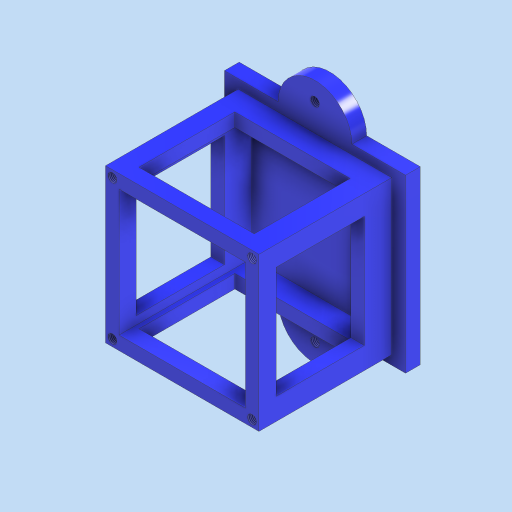
# Autodesk Inventor part: Base para Driver Corregida
Saved by Autodesk Inventor 2024 (Build 280153000, 153)
## iProperties
Created: 2023-12-03
Part Number: Base para Driver Corregida
Material: Genérico
Document SubType Name: Modeling
Designer: R3PT1L
Density: 1 g/cm^3
Appearance: Valor por defecto
Author: R3PT1L
Autodesk Inventor part; units mm, degrees
ref_plane "YZ Plane" through (0, 0, 0) normal (1, 0, 0) x (0, 1, 0)
ref_plane "XZ Plane" through (0, 0, 0) normal (0, 1, 0) x (-1, 0, 0)
ref_plane "XY Plane" through (0, 0, 0) normal (0, 0, 1) x (1, 0, 0)
sketch "Boceto1" plane through (0, 0, 0) normal (0, 0, 1) x (1, 0, 0)
  line L0 (-26, -26) -> (26, -26)
  line L1 (26, -26) -> (26, 26)
  line L2 (26, 26) -> (-26, 26)
  line L3 (-26, 26) -> (-26, -26)
  line L4 (-26, -26) -> (26, 26) construction
  line L5 (26, -26) -> (-26, 26) construction
  circle A0 centre (-23.6478, 23.6478) radius 1.5
  circle A1 centre (23.6478, 23.6478) radius 1.5
  circle A2 centre (23.6478, -23.6478) radius 1.5
  line L6 (-21.4311, -21.4311) -> (21.4311, -21.4311)
  line L7 (21.4311, -21.4311) -> (21.4311, 21.4311)
  line L8 (21.4311, 21.4311) -> (-21.4311, 21.4311)
  line L9 (-21.4311, 21.4311) -> (-21.4311, -21.4311)
  line L10 (-21.4311, -21.4311) -> (21.4311, 21.4311) construction
  line L11 (21.4311, -21.4311) -> (-21.4311, 21.4311) construction
  circle A3 centre (-23.6478, -23.6478) radius 1.5
  point P0 (0, 0)
  dimension "d0" = 52
  dimension "d1" = 52
  dimension "d2" = 3
  dimension "d3" = 3
  dimension "d4" = 3
  dimension "d6" = 3
  constraints: 24 end point, 5 point on line, 4 centre point, 4 midpoint, 4 parallel, 2 horizontal, 2 perpendicular
  measures "d0" distance of L2.end L1.end
  measures "d1" distance of L1.end L0.end
  measures "d2" diameter of A0
  measures "d3" diameter of A1
  measures "d4" diameter of A2
  measures "d6" diameter of A3
extrude "Extrusión1" add sketch "Boceto1" along normal blind 45
sketch "Boceto2" plane through (0, 0, 0) normal (0, 0, -1) x (-1, 0, 0)
  line L0 (30.6977, 29.0649) -> (-30.6977, 29.0649)
  line L1 (-30.6977, 29.0649) -> (-30.6977, -29.0649)
  line L2 (-30.6977, -29.0649) -> (30.6977, -29.0649)
  line L3 (30.6977, -29.0649) -> (30.6977, 29.0649)
  line L4 (30.6977, 29.0649) -> (-30.6977, -29.0649) construction
  line L5 (-30.6977, 29.0649) -> (30.6977, -29.0649) construction
  point P0 (0, 0)
  constraints: 12 end point, 2 midpoint, 2 parallel, 1 horizontal, 1 perpendicular
extrude "Extrusión2" add sketch "Boceto2" along normal blind 5
thread "Rosca1" size "M3x0.5" class "6H" standard "ANSI Metric M Profile" length 5
thread "Rosca2" size "M3x0.5" class "6H" standard "ANSI Metric M Profile" length 5
thread "Rosca3" size "M3x0.5" class "6H" standard "ANSI Metric M Profile" length 5
thread "Rosca4" size "M3x0.5" class "6H" standard "ANSI Metric M Profile" length 5
sketch "Boceto3" plane through (0, 0, -5) normal (0, 0, -1) x (-1, 0, 0)
  line L0 (-30.6977, -29.0649) -> (30.6977, -29.0649) projected
  arc A0 (-12.5, -29.0649) -> (12.5, -29.0649) centre (0, -29.0649) ccw
  line L1 (30.6977, 29.0649) -> (-30.6977, 29.0649) projected
  arc A1 (12.5, 29.0649) -> (-12.5, 29.0649) centre (0, 29.0649) ccw
  circle A2 centre (0, -35.3149) radius 1.5
  circle A3 centre (0, 35.3149) radius 1.5
  point P0 (0, 0)
  dimension "d19" = 25
  dimension "d20" = 25
  dimension "d21" = 3
  dimension "d22" = 3
  constraints: 4 centre point, 4 point on circle, 4 point on line, 2 midpoint
  measures "d19" diameter of A0
  measures "d20" diameter of A1
  measures "d21" diameter of A2
  measures "d22" diameter of A3
extrude "Extrusión3" add sketch "Boceto3" against normal blind 5
thread "Rosca5" size "M3x0.5" class "6H" standard "ANSI Metric M Profile" length 5
thread "Rosca6" size "M3x0.5" class "6H" standard "ANSI Metric M Profile" length 5
sketch "Boceto4" plane through (26, -26, 45) normal (1, 0, 0) x (0, 0, -1)
  line L0 (5.7927, 7.3891) -> (35.7255, 7.3891)
  line L1 (35.7255, 7.3891) -> (35.7255, 45.2774)
  line L2 (35.7255, 45.2774) -> (5.7927, 45.2774)
  line L3 (5.7927, 45.2774) -> (5.7927, 7.3891)
  point P0 (45, 26)
  constraints: 8 end point, 2 parallel, 1 horizontal, 1 perpendicular
extrude "Extrusión4" cut sketch "Boceto4" against normal blind 66
sketch "Boceto5" plane through (-26, 26, 45) normal (0, 1, 0) x (1, 0, 0)
  line L0 (45.1937, 5.2117) -> (6.1058, 5.2117)
  line L1 (6.1058, 5.2117) -> (6.1058, 37.7148)
  line L2 (6.1058, 37.7148) -> (45.1937, 37.7148)
  line L3 (45.1937, 37.7148) -> (45.1937, 5.2117)
  point P0 (26, 45)
  constraints: 8 end point, 2 parallel, 1 horizontal, 1 perpendicular
extrude "Extrusión5" cut sketch "Boceto5" against normal blind 66
